J7 (Autodesk Fusion 360 design; units mm, degrees)
part number: 2026-05-31-10-27-19-086
Autodesk Fusion 360 part; units mm, degrees
note: some values were not read from the file. Chosen so that the rebuilt part matches the saved one: that a step has no effect.
sketch "Sketch1" plane through (0, 0, 0) normal (0, 0, 1) x (1, 0, 0)
  line L0 (0, 0) -> (70, 0)
  line L1 (70, 0) -> (70, 40)
  line L2 (70, 40) -> (0, 40)
  line L3 (0, 40) -> (0, 0)
  circle A0 centre (15, 5) radius 1.25
  circle A1 centre (15, 30) radius 1.25
  circle A2 centre (45, 30) radius 1.25
  circle A3 centre (46, 5) radius 1.25
  dimension "d1" = 70
  dimension "d2" = 40
  dimension "d3" = 2.5
  dimension "d4" = 2.5
  dimension "d5" = 2.5
  dimension "d6" = 2.5
  constraint horizontal L0
  constraint vertical L1
  constraint horizontal L2
  constraint vertical L3
  constraint coincident L0.start L3.end
  measures "d1" distance of L0.start L0.end
  measures "d2" distance of L0.start L2.end
  measures "d3" diameter of A0
  measures "d4" diameter of A1
  measures "d5" diameter of A2
  measures "d6" diameter of A3
sketch "Sketch2" plane through (70, 0, 0) normal (1, 0, 0) x (0, 1, 0)
  line L0 (0, 0) -> (40, 0)
  line L1 (40, 0) -> (40, 40.2)
  line L2 (40, 40.2) -> (0, 40.2)
  line L3 (0, 40.2) -> (0, 0)
  circle A0 centre (20, 20) radius 15.1
  dimension "d9" = 30.2
  measures "d9" diameter of A0
sketch "Sketch3" plane through (70, 0, 0) normal (1, 0, 0) x (0, 1, 0)
  circle A0 centre (20, 20) radius 15.1
  line L0 (0, 0) -> (40, 0)
  line L1 (40, 0) -> (40, 40.2)
  line L2 (40, 40.2) -> (0, 40.2)
  line L3 (0, 40.2) -> (0, 0)
  circle A1 centre (20, 20) radius 19.1
  line L4 (0, 20.1) -> (0.9003, 20.1)
  line L5 (0.9003, 20.1) -> (0, 20.1)
  line L6 (0, 0) -> (40, 0)
  line L7 (40, 20.1) -> (40, 0)
  line L8 (40, 20) -> (39.1, 20)
  line L9 (39.1, 20) -> (40, 20)
  dimension "d12" = 38.2
  constraint concentric A0 A1
  constraint midpoint L3 L4.start
  constraint coincident A1 L4.end
  constraint perpendicular L3 L4
  constraint coincident L0.start L3.end
  constraint coincident L0.end L1.start
  constraint midpoint L1 L7.start
  constraint coincident L1 L8.start
  constraint coincident A1 L8.end
  constraint perpendicular L1 L8
  measures "d12" diameter of A1
sketch "Sketch4" plane through (0, 0, 40.2) normal (0, 0, 1) x (-1, 0, 0)
  circle A0 centre (-46, -5) radius 1.25
  circle A1 centre (-15, -5) radius 1.25
  circle A2 centre (-15, -30) radius 1.25
  circle A3 centre (-45, -30) radius 1.25
  line L0 (0, -40) -> (0, 0)
  line L1 (0, 0) -> (-70, 0)
  line L2 (-70, 0) -> (-70, -40)
  line L3 (-70, -40) -> (0, -40)
  circle A4 centre (-46, -5) radius 1.25
  constraint concentric A0 A4
sketch "Sketch5" plane through (0, 0, 40.2) normal (0, 0, 1) x (-1, 0, 0)
  circle A0 centre (-45, -5) radius 1.25
  circle A1 centre (-45, -5) radius 1.75
  circle A2 centre (-46, -5) radius 1.25
  dimension "d17" = 2.5
  dimension "d18" = 3.5
  constraint concentric A0 A1
  measures "d17" diameter of A0
  measures "d18" diameter of A1
sketch "Sketch6" plane through (0, 0, 40.2) normal (0, 0, 1) x (-1, 0, 0)
  arc A0 (-45.5, -3.8544) -> (-45.5, -6.1456) centre (-45, -5) ccw
  arc A1 (-45.5, -3.8544) -> (-45.5, -6.1456) centre (-46, -5) ccw
sketch "Sketch7" plane through (0, 0, 0) normal (1, 0, 0) x (0, 1, 0)
  circle A0 centre (20, 20) radius 15.1
  dimension "d25" = 30.2
  measures "d25" diameter of A0
sketch "Sketch8" plane through (0, 0, 40.2) normal (0, 0, 1) x (-1, 0, 0)
extrude "Extrude9" [no effect]
extrude "Extrude10" [no effect]
sketch "Sketch9" plane through (0, 0, 40.2) normal (0, 0, 1) x (-1, 0, 0)
sketch "Sketch10" plane through (0, 0, 40.2) normal (0, 0, 1) x (-1, 0, 0)
  circle A0 centre (-45, -30) radius 1.25
sketch "Sketch11" plane through (0, 0, 0) normal (0, 0, 1) x (1, 0, 0)
  line L0 (0, 0) -> (-60, 0)
  line L1 (-60, 0) -> (-60, -40)
  line L2 (-60, -40) -> (0, -40)
  line L3 (0, -40) -> (0, 0)
  dimension "d44" = 60
  dimension "d45" = 40
  constraint horizontal L0
  constraint vertical L1
  constraint horizontal L2
  constraint vertical L3
  constraint coincident L0.start L3.end
  measures "d44" distance of L0.start L0.end
  measures "d45" distance of L0.start L2.end
extrude "Extrude13" add sketch "Sketch11" along normal blind 42.2 makes body 1
sketch "Sketch12" plane through (-60, 0, 0) normal (-1, 0, 0) x (0, -1, 0)
  line L0 (0, 0) -> (40, 0)
  line L1 (40, 0) -> (40, 42.2)
  line L2 (40, 42.2) -> (0, 42.2)
  line L3 (0, 42.2) -> (0, 0)
  circle A0 centre (20, 20) radius 19.9392
  circle A1 centre (20, 20) radius 15.2
  line L4 (0, 20) -> (0, 0)
  line L5 (0, 0) -> (40, 0)
  line L6 (40, 0) -> (40, 21.1)
  line L7 (0, 20) -> (0.0608, 20)
  line L8 (40, 20) -> (39.9392, 20)
  dimension "d48" = 30.4
  constraint concentric A0 A1
  constraint coincident L3 L4.start
  constraint coincident L0.start L3.end
  constraint coincident L0.end L1.start
  constraint midpoint L1 L6.end
  constraint coincident A0 L7.end
  constraint perpendicular L4 L7
  constraint coincident L6 L8.start
  constraint coincident A0 L8.end
  constraint perpendicular L6 L8
  measures "d48" diameter of A1
extrude "Extrude14" cut sketch "Sketch12" against normal blind 60 contours L0 L1 L3 A0 L4 L5 L6 L7 L8 | A1 bodies 1
extrude "Extrude15" add 1 faces at (-60, -19.6214, 39.8525) along direction (-1, 0, 0) blind 5 on bodies 1 bodies 1
copy_body "CopyPasteBodies2" bodies 1 makes body 2
move_body "Move2" bodies 2 to x (0.819152, 0, -0.573576) y (0, 1, 0) z (0.573576, 0, 0.819152) at (29.2048, 0, -29.4415)
sketch "Sketch13" plane through (33.4297, 0, -23.4077) normal (0.819152, 0, -0.573576) x (0, 1, 0)
  line L0 (-0.0608, 12.6342) -> (0, 12.6342)
  line L1 (0, 12.6342) -> (0, 34.8342)
  line L2 (0, 34.8342) -> (-40, 34.8342)
  line L3 (-40, 34.8342) -> (-40, 12.6342)
  line L4 (-40, 12.6342) -> (-39.9392, 12.6342)
  arc A0 (-39.9392, 12.6342) -> (-0.0608, 12.6342) centre (-20, 12.6342) ccw
  circle A1 centre (-20, 12.6342) radius 15.2
  circle A2 centre (-20, 12.6342) radius 15.2
  constraint concentric A0 A2
extrude "Extrude16" cut sketch "Sketch13" against normal blind 65 contours A1 A2 bodies 1
sketch "Sketch14" plane through (-65, 0, 0) normal (-1, 0, 0) x (0, -1, 0)
  line L0 (0, 20) -> (0.0608, 20)
  arc A0 (0.0608, 20) -> (39.9392, 20) centre (20, 20) ccw
  line L1 (39.9392, 20) -> (40, 20)
  line L2 (40, 20) -> (40, 42.2)
  line L3 (40, 42.2) -> (0, 42.2)
  line L4 (0, 42.2) -> (0, 20)
  circle A1 centre (20, 20) radius 15.2
  circle A2 centre (20, 20) radius 15.2
  constraint concentric A0 A2
extrude "Extrude17" cut sketch "Sketch14" against normal blind 65 contours A1 A2 bodies 2
sketch "Sketch15" plane through (0, 0, 42.2) normal (0, 0, 1) x (-1, 0, 0)
  line L0 (0, 40) -> (0, 0)
  line L1 (0, 0) -> (65, 0)
  line L2 (65, 0) -> (65, 40)
  line L3 (65, 40) -> (0, 40)
  circle A0 centre (18, 5) radius 1.25
  circle A1 centre (18, 30) radius 1.25
  circle A2 centre (48, 30) radius 1.25
  circle A3 centre (48, 5) radius 1.25
  dimension "d58" = 2.5
  dimension "d60" = 2.5
  dimension "d61" = 30
  dimension "d62" = 2.5
  dimension "d63" = 30
  dimension "d64" = 2.5
  measures "d58" diameter of A0
  measures "d60" diameter of A1
  measures "d61" distance of A1.centre A2.centre
  measures "d62" diameter of A2
  measures "d63" distance of A0.centre A3.centre
  measures "d64" diameter of A3
extrude "Extrude18" cut sketch "Sketch15" against normal blind 60 contours A0 | A1 | A2 | A3 bodies 1 2
sketch "Sketch16" plane through (19.98, 0, 28.5345) normal (0.573576, 0, 0.819152) x (0, 1, 0)
  line L0 (-40, -40.8101) -> (0, -40.8101)
  line L1 (0, -40.8101) -> (0, 24.1899)
  line L2 (0, 24.1899) -> (-40, 24.1899)
  line L3 (-40, 24.1899) -> (-40, -40.8101)
  circle A0 centre (-5, 9) radius 1.25
  circle A1 centre (-35, 9) radius 1.25
  circle A2 centre (-35, -21) radius 1.25
  circle A3 centre (-5, -21) radius 1.25
  dimension "d67" = 2.5
  dimension "d68" = 2.5
  dimension "d69" = 30
  dimension "d70" = 2.5
  dimension "d71" = 2.5
  measures "d67" diameter of A0
  measures "d68" diameter of A1
  measures "d69" distance of A1.centre A2.centre
  measures "d70" diameter of A2
  measures "d71" diameter of A3
sketch "Sketch17" plane through (19.98, 0, 28.5345) normal (0.573576, 0, 0.819152) x (0, 1, 0)
  circle A0 centre (-30, 9) radius 1.25
  circle A1 centre (-30, -21) radius 1.25
  dimension "d72" = 2.5
  dimension "d73" = 2.5
  measures "d72" diameter of A0
  measures "d73" diameter of A1
sketch "Sketch18" plane through (19.98, 0, 28.5345) normal (0.573576, 0, 0.819152) x (0, 1, 0)
  circle A0 centre (-30, -21) radius 1.25
  dimension "d74" = 2.5
  measures "d74" diameter of A0
extrude "Extrude19" cut sketch "Sketch16" against normal blind 60 contours A0 | A1 | A2 | A3 bodies 1 2
sketch "Sketch19" plane through (0, 0, 42.2) normal (0, 0, 1) x (-1, 0, 0)
  circle A0 centre (18, 30) radius 1.25
  circle A1 centre (48, 30) radius 1.25
  circle A2 centre (18, 5) radius 1.25
  circle A3 centre (48, 5) radius 1.25
  line L0 (0, 40) -> (0, 0)
  line L1 (0, 0) -> (65, 0)
  line L2 (65, 0) -> (65, 40)
  line L3 (65, 40) -> (0, 40)
  circle A4 centre (48, 35) radius 1.25
  circle A5 centre (18, 35) radius 1.25
  dimension "d77" = 2.5
  dimension "d78" = 2.5
  measures "d77" diameter of A4
  measures "d78" diameter of A5
extrude "Extrude20" cut sketch "Sketch19" against normal blind 60 contours A4 | A5 bodies 1 2
